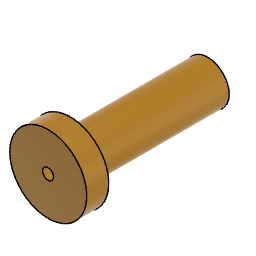
Back Hand Top Assembly v2 v7 (Autodesk Fusion 360 archive; units mm, degrees)
design "Pucks squeezer"
Autodesk Fusion 360 part; units mm, degrees
sketch "Base" plane through (0, 0, 0) normal (0, 1, 0) x (1, 0, 0)
  circle A0 centre (0, 0) radius 7
  dimension "d1" = 14
  constraint coincident A0.centre origin
  measures "d1" diameter of A0
extrude "Extrude1" add sketch "Base" along normal blind 4
sketch "Pin" plane through (0, 4, 0) normal (0, 1, 0) x (-1, 0, 0)
  circle A0 centre (0, 0) radius 7
  circle A1 centre (0, 0) radius 3.9
  dimension "d4" = 7.8
  constraint coincident A0.centre A1.centre
  measures "d4" diameter of A1
extrude "Extrude2" add sketch "Pin" along normal blind 25 contours A1
hole "Hole1" at (-0.0382, 0, -0.0078) direction (0, 1, 0) diameter 2 end through all

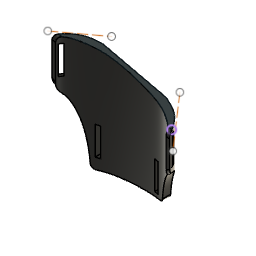
design "Back Hand Exo v4"
Autodesk Fusion 360 part; units mm, degrees
sketch "Base" plane through (0, 0, 0) normal (0, 0, 1) x (1, 0, 0)
  spline S0 degree 5 poles (13.752, -0.0001) (13.9653, 0.7958) (14.5381, 2.2842) (15.837, 4.206) (18.3493, 6.2617) (22.4599, 8.449) (27.2985, 10.6406) (33.3248, 12.6283) (41.3156, 13.6872) (50.5233, 13.835) (59.8574, 13.2455) (67.9918, 12.2717) (74.1601, 11.1616) (78.0856, 10.0513) (81.6903, 8.4944) (86.1249, 6.1568) (89.3627, 3.8311) (90.983, 1.9475) (91.5765, 0.6553) (91.752, 0) knots 0 0 0 0 0 0 0.066667 0.133333 0.2 0.266667 0.333333 0.4 0.466667 0.533333 0.6 0.666667 0.733333 0.8 0.866667 0.933333 1 1 1 1 1 1
  line L0 (11.7287, -7.5513) -> (15.7754, 7.551)
  line L1 (0, 0) -> (130, 0) construction
  line L2 (90.0188, 6.4684) -> (93.4853, -6.4684)
  line L3 (72.0197, 12) -> (83.6365, 8)
  line L4 (20.3175, 8.0956) -> (37.1866, 13.9041)
  line L5 (28.752, 32.4834) -> (28.752, -47.2676) construction
  line L6 (79.3904, 33.3073) -> (79.3904, -47.7619) construction
  line L7 (13.752, -0.0001) -> (11.252, 0)
  line L8 (94.252, 0) -> (91.752, 0)
  line L9 (30.252, 16.6538) -> (75.252, 16.6538)
  line L10 (52.752, 16.6538) -> (52.752, -22.3142) construction
  spline S1 degree 5 poles (11.252, 0) (11.5338, 0.5886) (12.1054, 1.7418) (12.9869, 3.3999) (14.2112, 5.465) (15.8292, 7.788) (17.544, 9.832) (19.3661, 11.5801) (21.3048, 13.0286) (23.3626, 14.2079) (25.537, 15.1728) (27.3674, 15.819) (28.7903, 16.2536) (29.7611, 16.5237) (30.252, 16.6538) knots 0 0 0 0 0 0 0.1 0.2 0.3 0.4 0.5 0.6 0.7 0.8 0.9 1 1 1 1 1 1
  spline S2 degree 5 poles (75.252, 16.6538) (75.631, 16.4987) (76.3973, 16.1962) (77.5715, 15.7657) (79.1807, 15.218) (81.2306, 14.4657) (83.2776, 13.5113) (85.2833, 12.2312) (87.2246, 10.5613) (89.093, 8.4929) (90.8878, 6.0413) (92.267, 3.7932) (93.2711, 1.9548) (93.9273, 0.6627) (94.252, 0) knots 0 0 0 0 0 0 0.1 0.2 0.3 0.4 0.5 0.6 0.7 0.8 0.9 1 1 1 1 1 1
  line L11 (26.8617, 15.7552) -> (33.6424, 17.5524)
  line L12 (72.1212, 17.9353) -> (78.3829, 15.3723)
  point P0 (28.752, 10.9999)
  point P1 (77.8281, 10)
  point P2 (20, 12)
  point P3 (84, 13)
  dimension "d1" = 78
  dimension "d3" = 15
  dimension "d4" = 11
  dimension "d5" = 10
  dimension "d6" = 75
  dimension "d7" = 75
  dimension "d8" = 19
  dimension "d9" = 19
  dimension "d10" = 2.5
  dimension "d11" = 2.5
  dimension "d71" = 45
  dimension "d72" = 39
  constraint midpoint S0.start L0
  constraint coincident L1.start origin
  constraint horizontal L1
  constraint midpoint S0.end L2
  constraint midpoint P1 L3
  constraint midpoint P0 L4
  constraint coincident L1 L7.end
  constraint coincident L1 L8.start
  constraint perpendicular L1 L5
  constraint vertical L6
  constraint coincident P0 L5
  constraint coincident S0.end L1
  constraint perpendicular L5 L9
  constraint vertical L10
  constraint midpoint L9 L10.start
  constraint midpoint L9.start L11
  constraint midpoint L9.end L12
  measures "d1" distance of S0.start S0.end
  measures "d3" distance of S0.start P0
  measures "d4" distance of S0.start P0
  measures "d5" distance of P1 S0.end
  measures "d6" angle of L0 L1
  measures "d7" angle of L1 L2
  measures "d8" angle of L1 L3
  measures "d9" angle of L1 L4
  measures "d10" distance of S0.end L8.start
  measures "d11" distance of S0.start L7.end
  measures "d71" distance of L9.start L9.end
  measures "d72" distance of S0.start L10
extrude "Extrude1" add sketch "Base" along normal blind 80
ref_plane "WorkPlane1" through (0, 34, 0) normal (0, 1, 0) x (0, 0, 1)
ref_plane "WorkPlane2" through (0, -2, 0) normal (0, 1, 0) x (0, 0, 1)
sketch "Bottom cut" plane through (0, -2, 0) normal (0, 1, 0) x (1, 0, 0)
  line L0 (104.8084, -94.0595) -> (104.8084, 16.0436) construction
  line L1 (124.2592, 0) -> (-25.481, 0) construction
  line L2 (7.8084, -95.0569) -> (7.8084, 27.3148) construction
  line L3 (10.7244, 0) -> (10.7244, -80) construction
  line L4 (100.7244, 0) -> (100.7244, -80) construction
  line L5 (-40, -55.0042) -> (-40, 40)
  line L6 (-40, 40) -> (120, 40)
  line L7 (120, 40) -> (120, -40)
  line L8 (120, -40) -> (104.8084, -39.0079)
  spline S0 degree 5 poles (4.5707, -55.0042) (5.4547, -54.2774) (7.185, -52.7903) (9.6672, -50.4587) (12.7463, -47.1447) (16.1864, -42.6382) (19.185, -37.7387) (21.7128, -32.42) (23.7655, -26.6781) (25.3732, -20.5401) (26.5747, -14.0405) (27.2401, -8.5774) (27.5837, -4.3416) (27.7449, -1.4573) (27.8084, 0) knots 0 0 0 0 0 0 0.1 0.2 0.3 0.4 0.5 0.6 0.7 0.8 0.9 1 1 1 1 1 1
  spline S1 degree 5 poles (104.8084, -39.0079) (103.8636, -38.7543) (102.0133, -38.2112) (99.3558, -37.2887) (96.0521, -35.8397) (92.3487, -33.6388) (89.108, -31.015) (86.3653, -27.9361) (84.1353, -24.3885) (82.3927, -20.3954) (81.0985, -15.9925) (80.3914, -12.1701) (80.0338, -9.1455) (79.871, -7.06) (79.8084, -6) knots 0 0 0 0 0 0 0.1 0.2 0.3 0.4 0.5 0.6 0.7 0.8 0.9 1 1 1 1 1 1
  line L9 (79.8084, -6) -> (27.8084, 0)
  line L10 (4.5707, -55.0042) -> (-40, -55.0042)
  point P0 (20.8084, -34.1255)
  point P1 (86.8084, -28.2303)
  dimension "d50" = 20
  dimension "d51" = 13
  dimension "d52" = 18
  dimension "d53" = 25
  dimension "d54" = 97
  dimension "d55" = 6
  constraint vertical L0
  constraint perpendicular L0 L1
  constraint perpendicular L1 L2
  constraint coincident origin L1
  constraint coincident L0 L8.end
  constraint perpendicular L5 L6
  constraint perpendicular L6 L7
  constraint vertical L5
  constraint perpendicular L5 L10
  constraint coincident L1 S0.end
  constraint midpoint L0 L8.end
  measures "d50" distance of L2 S0.end
  measures "d51" distance of L2 P0
  measures "d52" distance of L0 P1
  measures "d53" distance of L0 S1.end
  measures "d54" distance of L0 L2
  measures "d55" distance of L1 S1.end
sketch "Top cut" plane through (0, -2, 0) normal (0, 1, 0) x (1, 0, 0)
  line L0 (101.7244, -58) -> (2.8084, -81)
  line L1 (2.8084, -81) -> (2.8084, -105)
  line L2 (2.8084, -105) -> (101.7244, -105)
  line L3 (101.7244, -105) -> (101.7244, -58)
  line L4 (100.7244, -80) -> (10.7244, -80)
  line L5 (7.8084, -95.0569) -> (7.8084, 27.3148)
  line L6 (100.7244, 0) -> (100.7244, -80)
  dimension "d41" = 22
  dimension "d42" = 1
  dimension "d43" = 5
  dimension "d44" = 25
  dimension "d49" = 1
  constraint vertical L1
  constraint perpendicular L1 L2
  constraint perpendicular L2 L3
  measures "d41" distance of L0.start L4
  measures "d42" distance of L0.end L4
  measures "d43" distance of L1 L5
  measures "d44" distance of L2 L4
  measures "d49" distance of L3 L6
extrude "Extrude4" cut sketch "Bottom cut" along normal blind 40
extrude "Extrude5" cut sketch "Top cut" along normal blind 55
fillet "Fillet5" radius 3 6 edges at (27.8084, 13.3008, 0) (79.8084, 12.1091, 6) (12.502, -0.0001, 78.746) (93.002, 0, 60.0281) (12.5265, -0.0001, 47.1929) (92.9812, 0, 33.8848)
sketch "Strap holes1-2" plane through (0, 16.6538, 0) normal (0, 1, 0) x (-1, 0, 0)
  spline S0 degree 3 poles (-30.252, 0.3696) (-30.2872, 0.3651) (-30.3224, 0.3613) (-30.5631, 0.3393) (-30.7699, 0.3417) (-30.9749, 0.3654) knots 0.051258 0.051258 0.051258 0.051258 0.061889 0.061889 0.123778 0.123778 0.123778 0.123778
  line L0 (-30.252, 0.3696) -> (-30.252, 74.6188)
  line L1 (-30.252, 74.6188) -> (-75.252, 64.1554)
  line L2 (-75.252, 64.1554) -> (-75.252, 5.4743)
  line L3 (-75.252, 5.4743) -> (-30.9749, 0.3654)
  line L4 (-75.252, 28) -> (-72.252, 28)
  line L5 (-72.252, 28) -> (-72.252, 8)
  line L6 (-72.252, 8) -> (-75.252, 8)
  line L7 (-75.252, 8) -> (-75.252, 28)
  line L8 (-33.252, 28) -> (-30.252, 28)
  line L9 (-30.252, 28) -> (-30.252, 8)
  line L10 (-30.252, 8) -> (-33.252, 8)
  line L11 (-33.252, 8) -> (-33.252, 28)
  dimension "d86" = 20
  dimension "d87" = 8
  dimension "d88" = 8
  dimension "d89" = 3
  constraint horizontal L4
  constraint vertical L5
  constraint horizontal L6
  constraint vertical L7
  constraint horizontal L8
  constraint vertical L9
  constraint horizontal L10
  constraint vertical L11
  constraint equal L5 L9
  constraint equal L6 L10
  constraint collinear L2 L7
  constraint collinear L0 L9
  measures "d86" distance of L8.end L9.end
  measures "d87" distance of origin L6
  measures "d88" distance of origin L10
  measures "d89" distance of L8.start L8.end
extrude "Extrude9" cut sketch "Strap holes1-2" against normal blind 12 contours L0 L8 L9 L10 L11 | L2 L4 L5 L6 L7
sketch "Construction lines" plane through (18.0122, 0, 77.4648) normal (0.226479, 0, 0.974016) x (0, 1, 0)
  line L0 (3, -73.8013) -> (3, -76.6575)
  spline S0 degree 3 poles (16.6538, -58.7669) (15.8139, -60.8738) (15.3084, -62.6333) (13.7959, -66.4997) (12.7514, -68.5403) (8.7557, -72.9177) (6.0876, -74.8715) (3, -76.6575) knots -3.463321 -3.463321 -3.463321 -3.463321 -2.542901 -2.542901 -1.469021 -1.469021 -0.348561 -0.348561 -0.348561 -0.348561
  line L1 (16.6538, -58.7669) -> (16.6538, -12.5664)
  spline S1 degree 3 poles (3, 5.3518) (4.4398, 4.5288) (5.8451, 3.6285) (9.4992, 0.8936) (11.0843, -0.7862) (13.6108, -4.229) (15.2503, -7.1298) (16.6538, -12.5664) knots -3.904923 -3.904923 -3.904923 -3.904923 -3.114185 -3.114185 -1.684445 -1.684445 0 0 0 0
  line L2 (3, 5.3518) -> (2.9998, 2.9242)
  spline S2 degree 3 poles (3, -73.8013) (3.7027, -73.1055) (4.3459, -72.2992) (6.4441, -69.3508) (7.7722, -66.7548) (9.2291, -63.5462) (9.772, -62.1746) (12.4028, -53.6965) (13.5824, -40.3684) (13.809, -19.6639) (12.0211, -13.2463) (9.1223, -6.1584) (7.6302, -2.7127) (5.085, 0.9851) (4.2261, 1.9685) (3.156, 2.8074) (3.0782, 2.8665) (2.9998, 2.9242) knots -6.903103 -6.903103 -6.903103 -6.903103 -6.723866 -6.723866 -6.232481 -6.232481 -5.876872 -5.876872 -4.173273 -4.173273 -1.579181 -1.579181 -0.749477 -0.749477 -0.371417 -0.371417 -0.342017 -0.342017 -0.342017 -0.342017
  line L3 (0, 10) -> (24.0161, -11.5563) construction
  line L4 (25, -60) -> (-7.1736, -87.8504) construction
ref_plane "WorkPlane3" through (18.7701, 12.0081, 77.2886) normal (0.752855, -0.658187, 0) x (0.650612, 0.74419, -0.151281)
ref_plane "WorkPlane4" through (90.0165, 8.9132, 60.7223) normal (-0.764523, -0.644597, 0) x (0.637476, -0.756077, -0.148226)
sketch "Strap hole3" plane through (18.7701, 12.0081, 77.2886) normal (0.752855, -0.658187, 0) x (0.650612, 0.74419, -0.151281)
  line L0 (-16.1358, 0) -> (16.1358, 0)
  line L1 (-14.3189, 1.0938) -> (-8.2677, -38.4458) construction
  line L2 (-10.1527, -26.1289) -> (-13.6261, -3.4328) construction
  line L3 (-10.3799, -4.8256) -> (-7.3543, -24.5954)
  line L4 (-7.3543, -24.5954) -> (-4.3889, -24.1416)
  line L5 (-4.3889, -24.1416) -> (-7.4145, -4.3718)
  line L6 (-7.4145, -4.3718) -> (-10.3799, -4.8256)
  dimension "d97" = 40
  dimension "d98" = 20
  dimension "d99" = 3
  constraint parallel L1 L2
  constraint collinear L1 L2
  constraint parallel L1 L3
  constraint perpendicular L3 L4
  constraint perpendicular L3 L6
  constraint parallel L3 L5
  measures "d97" distance of L1.start L1.end
  measures "d98" distance of L3.start L3.end
  measures "d99" distance of L3.end L4.end
extrude "Extrude10" cut sketch "Strap hole3" along normal blind 15
sketch "Strap hole4" plane through (90.0165, 8.9132, 60.7223) normal (-0.764523, -0.644597, 0) x (0.637476, -0.756077, -0.148226)
  line L0 (8.5937, 7.0554) -> (14.6402, -33.2862) construction
  line L1 (12.7879, -20.9277) -> (10.0417, -2.6052) construction
  line L2 (6.0688, -3.0847) -> (9.0334, -22.8638)
  line L3 (6.0688, -3.0847) -> (3.102, -3.5294)
  line L4 (3.102, -3.5294) -> (6.0665, -23.3084)
  line L5 (6.0665, -23.3084) -> (9.0334, -22.8638)
  dimension "d102" = 20
  dimension "d103" = 4
  dimension "d104" = 4
  dimension "d105" = 3
  constraint collinear L0 L1
  constraint perpendicular L2 L3
  constraint perpendicular L3 L4
  constraint perpendicular L4 L5
  measures "d102" distance of L2.start L2.end
  measures "d103" distance of L0 L2.end
  measures "d104" distance of L0 L2.start
  measures "d105" distance of L2.start L3.end
extrude "Extrude11" cut sketch "Strap hole4" along normal blind 20
equation "d72 = ( 78 / 2 ) * 1 mm"

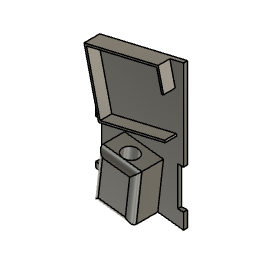
design "Back Hand Exo Top v1"
Autodesk Fusion 360 part; units mm, degrees
ref_plane "WorkPlane3" through (54.5653, 17.8993, 37.432) normal (0, 1, 0) x (-1, 0, 0)
sketch "Top part base" plane through (54.5653, 17.8993, 37.432) normal (0, 1, 0) x (1, 0, 0)
  line L0 (25.2893, -113.3578) -> (25.2893, -39.0578)
  line L1 (25.2893, -39.0578) -> (-19.7107, -44.2645)
  line L2 (-19.7107, -44.2645) -> (-19.7107, -102.7645)
  line L3 (-19.7107, -102.7645) -> (25.2893, -113.3578)
  line L4 (-30, 0) -> (100, 0) construction
  dimension "d112" = 45
  dimension "d113" = 58.5
  dimension "d114" = 74.3
  dimension "d115" = 6.6
  constraint vertical L0
  constraint parallel L0 L2
  constraint horizontal L4
  measures "d112" distance of L0 L2
  measures "d113" distance of L1.end L2.end
  measures "d114" distance of L0.start L0.end
  measures "d115" angle of L1 L4
extrude "Extrude9" add sketch "Top part base" along normal blind 2
sketch "Anchor" plane through (0, 17.8993, 0) normal (0, -1, 0) x (1, 0, 0)
  line L0 (79.8546, 150.7899) -> (34.8546, 140.1965)
  line L1 (34.8546, 140.1965) -> (34.8546, 81.6965)
  line L2 (34.8546, 81.6965) -> (79.8546, 76.4899)
  line L3 (79.8546, 76.4899) -> (79.8546, 150.7899)
  line L4 (11.5702, 84.3906) -> (87.0208, 75.6607) construction
  line L5 (46.7751, 80.3173) -> (66.6426, 78.0185)
  line L6 (66.6426, 78.0185) -> (69.516, 102.8529)
  line L7 (69.516, 102.8529) -> (49.6485, 105.1516)
  line L8 (49.6485, 105.1516) -> (46.7751, 80.3173)
  dimension "d86" = 90
  dimension "d87" = 90
  dimension "d88" = 90
  dimension "d89" = 12
  dimension "d90" = 20
  dimension "d91" = 25
  constraint collinear L2 L4
  constraint coincident L2 L5.start
  constraint coincident L4 L5.start
  constraint coincident L2 L5.end
  constraint perpendicular L6 L7
  measures "d86" angle of L5 L6
  measures "d87" angle of L5 L8
  measures "d88" angle of L7 L8
  measures "d89" distance of L1.end L5.start
  measures "d90" distance of L5.start L5.end
  measures "d91" distance of L5.end L6.end
extrude "Extrude10" add sketch "Anchor" along normal blind 14 contours L2 L5 L6 L7 L8
sketch "Stopper battery" plane through (0, 17.8993, 0) normal (0, -1, 0) x (1, 0, 0)
  line L0 (69.516, 102.8529) -> (66.6426, 78.0185)
  line L1 (66.6426, 78.0185) -> (79.8546, 76.4899)
  line L2 (79.8546, 76.4899) -> (79.8546, 150.7899)
  line L3 (79.8546, 150.7899) -> (34.8546, 140.1965)
  line L4 (34.8546, 140.1965) -> (34.8546, 81.6965)
  line L5 (34.8546, 81.6965) -> (46.7751, 80.3173)
  line L6 (46.7751, 80.3173) -> (49.6485, 105.1516)
  line L7 (49.6485, 105.1516) -> (69.516, 102.8529)
  line L8 (34.8546, 140.1965) -> (72.8169, 149.1331)
  line L9 (34.8546, 140.1965) -> (42.3018, 108.5613)
  line L10 (42.3018, 108.5613) -> (76.3705, 116.5813)
  line L11 (76.3705, 116.5813) -> (76.1414, 117.5547)
  line L12 (76.1414, 117.5547) -> (43.0461, 109.7638)
  line L13 (43.0461, 109.7638) -> (36.0572, 139.4523)
  line L14 (36.0572, 139.4523) -> (72.0727, 147.9306)
  line L15 (72.8169, 149.1331) -> (75.5667, 137.4524)
  line L16 (75.5667, 137.4524) -> (74.5933, 137.2233)
  line L17 (74.5933, 137.2233) -> (72.0727, 147.9306)
  dimension "d116" = 39
  dimension "d117" = 32.5
  dimension "d118" = 35
  dimension "d119" = 1
  dimension "d120" = 1
  dimension "d121" = 1
  dimension "d122" = 12
  dimension "d123" = 1
  dimension "d124" = 1
  constraint coincident L3.end L4.start
  constraint parallel L3 L8
  constraint perpendicular L3 L9
  constraint perpendicular L9 L10
  constraint perpendicular L10 L11
  constraint perpendicular L11 L12
  constraint perpendicular L12 L13
  constraint perpendicular L13 L14
  constraint perpendicular L3 L15
  constraint perpendicular L15 L16
  measures "d116" distance of L3.end L8.end
  measures "d117" distance of L3.end L9.end
  measures "d118" distance of L9.end L10.end
  measures "d119" distance of L10.end L11.end
  measures "d120" distance of L9 L13
  measures "d121" distance of L8 L14
  measures "d122" distance of L8.end L15.end
  measures "d123" distance of L15.end L16.end
  measures "d124" distance of L14.end L15
sketch "Anchor hole" plane through (9.7882, 0, 84.5968) normal (-0.114937, 0, -0.993373) x (0, 1, 0)
  line L0 (17.8993, 70.5339) -> (17.8993, 57.2337)
  line L1 (17.8993, 57.2337) -> (3.8993, 57.2337)
  line L2 (3.8993, 57.2337) -> (3.8993, 37.2337)
  line L3 (3.8993, 37.2337) -> (17.8993, 37.2337)
  line L4 (17.8993, 37.2337) -> (17.8993, 25.2337)
  line L5 (17.8993, 25.2337) -> (19.8993, 25.2337)
  line L6 (19.8993, 25.2337) -> (19.8993, 70.5339)
  line L7 (19.8993, 70.5339) -> (17.8993, 70.5339)
  circle A0 centre (10.8993, 47.2337) radius 4
  line L8 (19.8993, 47.2337) -> (3.8993, 47.2337) construction
  dimension "d109" = 8
  dimension "d110" = 7
  constraint perpendicular L2 L8
  constraint midpoint L2 L8.end
  constraint coincident A0.centre L8
  constraint coincident L6 L8.start
  measures "d109" diameter of A0
  measures "d110" distance of L2 A0.centre
hole "Hole3" at (56.7088, 10.8993, 79.1679) direction (0.114937, 0, 0.993373) diameter 8 end up to surface (25 mm away)
extrude "Extrude12" add sketch "Stopper battery" along normal blind 6 contours L3 L8 L9 L10 L11 L12 L13 L14 L15 L16 L17
sketch "Strap holes" plane through (0, 17.8993, 0) normal (0, -1, 0) x (1, 0, 0)
  line L0 (72.8169, 149.1331) -> (75.5667, 137.4524)
  line L1 (75.5667, 137.4524) -> (74.5933, 137.2233)
  line L2 (74.5933, 137.2233) -> (72.0727, 147.9306)
  line L3 (72.0727, 147.9306) -> (36.0572, 139.4523)
  line L4 (36.0572, 139.4523) -> (43.0461, 109.7638)
  line L5 (43.0461, 109.7638) -> (76.1414, 117.5547)
  line L6 (76.1414, 117.5547) -> (76.3705, 116.5813)
  line L7 (76.3705, 116.5813) -> (42.3018, 108.5613)
  line L8 (42.3018, 108.5613) -> (34.8546, 140.1965)
  line L9 (34.8546, 140.1965) -> (34.8546, 81.6965)
  line L10 (34.8546, 81.6965) -> (46.7751, 80.3173)
  line L11 (46.7751, 80.3173) -> (49.6485, 105.1516)
  line L12 (49.6485, 105.1516) -> (69.516, 102.8529)
  line L13 (69.516, 102.8529) -> (66.6426, 78.0185)
  line L14 (66.6426, 78.0185) -> (79.8546, 76.4899)
  line L15 (79.8546, 76.4899) -> (79.8546, 150.7899)
  line L16 (79.8546, 150.7899) -> (72.8169, 149.1331)
  line L17 (34.8546, 104.4899) -> (37.8546, 104.4899)
  line L18 (37.8546, 104.4899) -> (37.8546, 84.4899)
  line L19 (37.8546, 84.4899) -> (34.8546, 84.4899)
  line L20 (34.8546, 84.4899) -> (34.8546, 104.4899)
  line L21 (76.8546, 104.4899) -> (79.8546, 104.4899)
  line L22 (79.8546, 104.4899) -> (79.8546, 84.4899)
  line L23 (79.8546, 84.4899) -> (76.8546, 84.4899)
  line L24 (76.8546, 84.4899) -> (76.8546, 104.4899)
  dimension "d127" = 20
  dimension "d128" = 8
  dimension "d129" = 3
  constraint horizontal L17
  constraint vertical L18
  constraint horizontal L19
  constraint vertical L20
  constraint horizontal L21
  constraint vertical L22
  constraint horizontal L23
  constraint vertical L24
  constraint equal L18 L22
  constraint collinear L19 L23
  constraint equal L19 L23
  constraint collinear L15 L22
  constraint collinear L9 L20
  measures "d127" distance of L21.end L22.end
  measures "d128" vertical distance of L14.end L19.end
  measures "d129" distance of L22.end L23.end
extrude "Extrude13" cut sketch "Strap holes" against normal blind 10 contours L15 L21 L22 L23 L24 | L9 L17 L18 L19 L20
fillet "Fillet5" radius 3 4 edges at (59.5823, 3.8993, 104.0022) (68.0793, 3.8993, 90.4357) (48.2118, 3.8993, 92.7344) (56.7088, 3.8993, 79.1679)

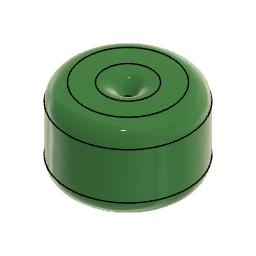
design "Puck_12 mm h"
Autodesk Fusion 360 part; units mm, degrees
sketch "Sketch1" plane through (0, 0, 0) normal (0, 0, 1) x (1, 0, 0)
  circle A0 centre (25, 25) radius 9
  circle A1 centre (25, 25) radius 1
  dimension "d1" = 18
  dimension "d2" = 2
  constraint concentric A0 A1
  measures "d1" diameter of A0
  measures "d2" diameter of A1
extrude "Extrude1" add sketch "Sketch1" along normal blind 12
fillet "Fillet1" radius 2.5 4 faces at (31.2961, 24.5032, 12) (25.7971, 25.6038, 8) (33.9888, 24.5514, 8) (31.2961, 24.5032, 0)

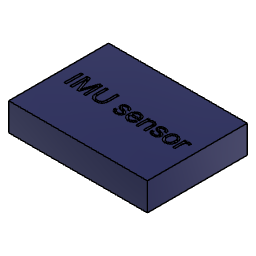
design "IMU sensor"
Autodesk Fusion 360 part; units mm, degrees
sketch "Sketch1" plane through (0, 0, 0) normal (0, 0, 1) x (1, 0, 0)
  line L0 (0, 0) -> (25, 0)
  line L1 (25, 0) -> (25, 18)
  line L2 (25, 18) -> (0, 18)
  line L3 (0, 18) -> (0, 0)
  dimension "d1" = 25
  dimension "d2" = 18
  constraint horizontal L0
  constraint vertical L1
  constraint horizontal L2
  constraint vertical L3
  constraint coincident L0.start L3.end
  measures "d1" distance of L0.start L0.end
  measures "d2" distance of L0.start L2.end
extrude "Extrude1" add sketch "Sketch1" along normal blind 5
sketch "Sketch2" plane through (0, 0, 5) normal (0, 0, 1) x (-1, 0, 0)
  line L0 (0, -18) -> (0, 0)
  line L1 (0, 0) -> (-25, 0)
  line L2 (-25, 0) -> (-25, -18)
  line L3 (-25, -18) -> (0, -18)
  line L4 (-2.096, -5.6815) -> (-24.9212, -5.335) construction
  line L5 (-24.9212, -5.335) -> (-25, -10.5236) construction
  line L6 (-25, -10.5236) -> (-2.1747, -10.87) construction
  line L7 (-2.1747, -10.87) -> (-2.096, -5.6815) construction
  dimension "d5" = 3
  text T0 "IMU sensor" font "Arial" height 3 align left top in box 22.8279 x 5.1892 at (-2.096, -5.6815) x (-0.999885, 0.015176) y (-0.015176, -0.999885) spacing 1 kerned
  constraint coincident L2
extrude "Extrude2" cut sketch "Sketch2" against normal blind 1 text T0
